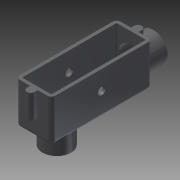
# Autodesk Inventor part: Access Fitting
Saved by Autodesk Inventor 2015 SP1 (Build 190203100, 203)
## iProperties
Created: 2015-02-01
Part Number: Access Fitting
Material: PVC-Piping
Document SubType Name: Modeling
Designer: Brian
Density: 1.4 g/cm^3
Appearance: Smooth - Medium Gray
Author: Brian
Autodesk Inventor part; units mm, degrees
ref_plane "YZ Plane" through (0, 0, 0) normal (1, 0, 0) x (0, 1, 0)
ref_plane "XZ Plane" through (0, 0, 0) normal (0, 1, 0) x (-1, 0, 0)
ref_plane "XY Plane" through (0, 0, 0) normal (0, 0, 1) x (1, 0, 0)
sketch "Sketch1" plane through (0, 0, 0) normal (0, 1, 0) x (-1, 0, 0)
  line L0 (-44.45, -5.08) -> (-44.45, -121.0737)
  line L1 (0, -121.0737) -> (0, -5.08)
  arc A0 (0, -5.08) -> (-5.08, 0) centre (-5.08, -5.08) ccw
  arc A1 (-39.37, 0) -> (-44.45, -5.08) centre (-39.37, -5.08) ccw
  arc A2 (-44.45, -121.0737) -> (-39.37, -126.1537) centre (-39.37, -121.0737) ccw
  arc A3 (-5.08, -126.1537) -> (0, -121.0737) centre (-5.08, -121.0737) ccw
  line L2 (-17.9596, 0) -> (-17.9596, 3.995)
  line L3 (-27.432, 0) -> (-27.432, 3.995)
  line L4 (-17.9596, -126.1537) -> (-17.9596, -130.1487)
  line L5 (-27.432, -126.1537) -> (-27.432, -130.1487)
  arc A4 (-17.9596, 3.995) -> (-27.432, 3.995) centre (-22.6958, 3.995) ccw
  arc A5 (-27.432, -130.1487) -> (-17.9596, -130.1487) centre (-22.6958, -130.1487) ccw
  line L6 (-5.08, 0) -> (-17.9596, 0)
  line L7 (-27.432, 0) -> (-39.37, 0)
  line L8 (-39.37, -126.1537) -> (-27.432, -126.1537)
  line L9 (-17.9596, -126.1537) -> (-5.08, -126.1537)
  point P0 (0, 0)
  point P1 (-44.45, -125.5501)
  point P2 (-44.45, 0)
  point P3 (0, -125.5501)
  point P4 (-22.6958, 8.7313)
  dimension "d1" = 44.45
  dimension "d2" = 5.08
  dimension "d6" = 134.1438
  dimension "d19" = 8.7312
  constraints: 20 end point, 14 tangent, 13 point on circle, 6 centre point, 5 parallel, 5 point on line, 4 equal radius, 4 vertical, 3 collinear, 2 horizontal, 2 horizontal alignment, 2 perpendicular
  measures "d1" distance of point (-44.45, -125.55) point (0, -125.55)
  measures "d2" radius of A0
  measures "d6" distance of A5.centre A4.centre
  measures "d19" distance from line of L7 point (-22.696, 8.731)
extrude "Extrusion1" add sketch "Sketch1" along normal blind 51.5938
sketch "Sketch4" plane through (0, 0, 0) normal (0, -1, 0) x (1, 0, 0)
  arc A0 (5.08, 0) -> (0, -5.08) centre (5.08, -5.08) ccw construction
  line L0 (0, -5.08) -> (0, -121.0737) construction
  arc A1 (0, -121.0737) -> (5.08, -126.1537) centre (5.08, -121.0737) ccw construction
  line L1 (5.08, -126.1537) -> (17.9596, -126.1537) construction
  line L2 (17.9596, -126.1537) -> (17.9596, -130.1487) construction
  arc A2 (17.9596, -130.1487) -> (27.432, -130.1487) centre (22.6958, -130.1487) ccw construction
  line L3 (27.432, -130.1487) -> (27.432, -126.1537) construction
  line L4 (27.432, -126.1537) -> (39.37, -126.1537) construction
  arc A3 (39.37, -126.1537) -> (44.45, -121.0737) centre (39.37, -121.0737) ccw construction
  line L5 (44.45, -121.0737) -> (44.45, -5.08) construction
  arc A4 (44.45, -5.08) -> (39.37, 0) centre (39.37, -5.08) ccw construction
  line L6 (39.37, 0) -> (27.432, 0) construction
  line L7 (27.432, 0) -> (27.432, 3.995) construction
  arc A5 (27.432, 3.995) -> (17.9596, 3.995) centre (22.6958, 3.995) ccw construction
  line L8 (17.9596, 3.995) -> (17.9596, 0) construction
  line L9 (17.9596, 0) -> (5.08, 0) construction
  circle A6 centre (22.6958, -28.5224) radius 17.8911
  point P0 (0, 0)
  dimension "d17" = 35.7822
  dimension "d18" = 97.6312
  constraints: 1 centre point, 1 vertical alignment
  measures "d17" diameter of A6
  measures "d18" distance from line of L4 A6.centre
extrude "Extrusion2" add sketch "Sketch4" along normal blind 23.8125
sketch "Sketch5" plane through (22.6958, -23.8125, -28.5224) normal (0, -1, 0) x (1, 0, 0)
  arc A0 (-17.6158, 28.5224) -> (-22.6958, 23.4424) centre (-17.6158, 23.4424) ccw construction
  line L0 (-22.6958, 23.4424) -> (-22.6958, -92.5512) construction
  arc A1 (-22.6958, -92.5512) -> (-17.6158, -97.6312) centre (-17.6158, -92.5512) ccw construction
  line L1 (-17.6158, -97.6312) -> (-4.7362, -97.6312) construction
  line L2 (-4.7362, -97.6312) -> (-4.7362, -101.6263) projected
  arc A2 (-4.7362, -101.6263) -> (4.7362, -101.6263) centre (0, -101.6263) ccw projected
  line L3 (4.7362, -101.6263) -> (4.7362, -97.6313) projected
  line L4 (4.7362, -97.6313) -> (16.6742, -97.6313) construction
  arc A3 (16.6742, -97.6313) -> (21.7542, -92.5512) centre (16.6742, -92.5512) ccw construction
  line L5 (21.7542, -92.5512) -> (21.7542, 23.4424) construction
  arc A4 (21.7542, 23.4424) -> (16.6742, 28.5224) centre (16.6742, 23.4424) ccw construction
  line L6 (16.6742, 28.5224) -> (4.7362, 28.5224) construction
  line L7 (4.7362, 28.5224) -> (4.7362, 32.5175) projected
  arc A5 (4.7362, 32.5175) -> (-4.7362, 32.5175) centre (0, 32.5175) ccw projected
  line L8 (-4.7362, 32.5175) -> (-4.7362, 28.5224) projected
  line L9 (-4.7362, 28.5224) -> (-17.6158, 28.5224) construction
  line L10 (4.7362, -97.6313) -> (-4.7362, -97.6312)
  line L11 (4.7362, 28.5224) -> (-4.7362, 28.5224)
  point P0 (-22.6958, 28.5224)
  constraints: 4 end point, 2 horizontal
extrude "Extrusion3" cut sketch "Sketch5" against normal blind 45.2437
sketch "Sketch6" plane through (39.37, 0, -126.1537) normal (0, 0, -1) x (-1, 0, 0)
  line L0 (0, 0) -> (0, 51.5938) construction
  line L1 (34.29, 0) -> (0, 0) construction
  line L2 (34.29, 0) -> (34.29, 51.5938) construction
  line L3 (0, 51.5938) -> (34.29, 51.5938) construction
  line L4 (21.4104, 51.5938) -> (34.29, 51.5938) construction
  circle A0 centre (17.145, 21.4312) radius 17.8911
  line L5 (-1.2169, -23.8125) -> (34.5653, -23.8125) construction
  point P0 (39.37, 0)
  dimension "d13" = 45.2437
  dimension "d14" = 35.7822
  constraints: 2 end point, 1 centre point, 1 collinear
  measures "d13" distance from line of L5 A0.centre
  measures "d14" diameter of A0
extrude "Extrusion4" add sketch "Sketch6" along normal blind 23.8125
sketch "Sketch7" plane through (0, 51.5938, 0) normal (0, 1, 0) x (1, 0, 0)
  line L0 (44.45, 5.08) -> (44.45, 121.0737) construction
  line L1 (0, 121.0737) -> (0, 5.08) construction
  arc A0 (5.08, 126.1537) -> (0, 121.0737) centre (5.08, 121.0737) ccw construction
  line L2 (5.08, 126.1537) -> (39.37, 126.1537) construction
  arc A1 (44.45, 121.0737) -> (39.37, 126.1537) centre (39.37, 121.0737) ccw construction
  arc A2 (39.37, 0) -> (44.45, 5.08) centre (39.37, 5.08) ccw construction
  line L3 (5.08, 0) -> (17.9596, 0) construction
  line L4 (27.432, 0) -> (39.37, 0) construction
  line L5 (27.432, 0) -> (17.9596, 0) construction
  arc A3 (0, 5.08) -> (5.08, 0) centre (5.08, 5.08) ccw construction
  line L6 (40.4812, 121.0737) -> (40.4812, 5.08)
  arc A4 (39.37, 3.9687) -> (40.4812, 5.08) centre (39.37, 5.08) ccw
  line L7 (39.37, 3.9687) -> (27.432, 3.9687)
  line L8 (27.432, 3.9687) -> (17.9596, 3.9687)
  line L9 (17.9596, 3.9687) -> (5.08, 3.9687)
  arc A5 (3.9688, 5.08) -> (5.08, 3.9687) centre (5.08, 5.08) ccw
  line L10 (3.9688, 5.08) -> (3.9687, 121.0737)
  arc A6 (5.08, 122.1849) -> (3.9687, 121.0737) centre (5.08, 121.0737) ccw
  line L11 (5.08, 122.1849) -> (39.37, 122.1849)
  arc A7 (40.4812, 121.0737) -> (39.37, 122.1849) centre (39.37, 121.0737) ccw
  point P0 (0, 0)
  dimension "d20" = 3.9688
  constraints: 12 end point, 8 point on circle, 4 centre point, 9 other
  measures "d20" distance between parallel lines of L0 L6
extrude "Extrusion5" cut sketch "Sketch7" against normal blind 47.625
sketch "Sketch8" plane through (22.6958, -23.8125, -28.5224) normal (0, -1, 0) x (1, 0, 0)
  circle A0 centre (0, 0) radius 17.8911 construction
  circle A1 centre (0, 0) radius 16.7005
  point P0 (-22.6958, 28.5224)
  dimension "d23" = 33.401
  constraints: 1 centre point, 1 coincident
  measures "d23" diameter of A1
extrude "Extrusion6" cut sketch "Sketch8" against normal up to surface (27.7812 mm away)
sketch "Sketch9" plane through (22.225, 21.4312, -149.9662) normal (0, 0, -1) x (-1, 0, 0)
  circle A0 centre (0, 0) radius 17.8911 construction
  circle A1 centre (0, 0) radius 16.7005
  point P0 (22.225, -21.4312)
  dimension "d26" = 33.401
  constraints: 1 centre point, 1 coincident
  measures "d26" diameter of A1
extrude "Extrusion7" cut sketch "Sketch9" against normal up to surface (27.7812 mm away)
sketch "Sketch10" plane through (5.08, 51.5938, -122.1849) normal (0, 0, 1) x (1, 0, 0)
  circle A0 centre (17.145, -30.1625) radius 16.7005 projected
  circle A1 centre (17.145, -30.1625) radius 15.9067
  point P0 (-5.08, -51.5938)
  dimension "d29" = 0.7937
  constraints: 1 centre point, 1 coincident
  measures "d29" radial gap between concentric circles of A0 A1
extrude "Extrusion8" add sketch "Sketch10" against normal blind 3.9688
sketch "Sketch11" plane through (0, 3.9687, 0) normal (0, 1, 0) x (1, 0, 0)
  circle A0 centre (22.6958, 28.5224) radius 16.7005 projected
  circle A1 centre (22.6958, 28.5224) radius 15.9067
  point P0 (0, 0)
  dimension "d32" = 0.7937
  constraints: 1 centre point, 1 coincident
  measures "d32" radial gap between concentric circles of A1 A0
extrude "Extrusion9" add sketch "Sketch11" against normal blind 3.9688
fillet "Fillet1" radius 3.175 9 edges at (1.4879, 0, -124.6658) (22.225, 0, -126.1537) (42.9621, 0, -124.6658) (44.45, 0, -63.0768) (42.9621, 0, -1.4879) (22.225, 0, 0) (1.4879, 0, -1.4879) (0, 0, -63.0768) (4.8047, 0, -28.5224)
sketch "Sketch12" plane through (44.45, 51.5938, -5.08) normal (1, 0, 0) x (0, 0, -1)
  line L0 (0, 0) -> (115.9937, 0) construction
  line L1 (0, 0) -> (0, -47.625) construction
  line L2 (0, -47.625) -> (115.9937, -47.625) construction
  line L3 (115.9937, 0) -> (115.9937, -47.625) construction
  circle A0 centre (57.9968, -23.8125) radius 4.7625
  point P0 (-5.08, -51.5938)
  point P1 (57.9968, 0)
  point P2 (0, -23.8125)
  dimension "d36" = 9.525
  constraints: 2 midpoint, 1 centre point, 1 horizontal alignment, 1 vertical alignment
  measures "d36" diameter of A0
extrude "Extrusion10" cut sketch "Sketch12" against normal up to surface (44.45 mm away)
body "Solid1"
